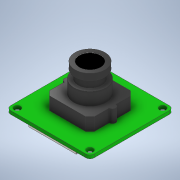
# Autodesk Inventor part: Innomaker_OV9281
Saved by Autodesk Inventor 2020 (Build 240168000, 168)
## iProperties
Created: 2021-04-16
Part Number: Innomaker_OV9281
Material: Generic
Document SubType Name: Modeling
Designer: junnu
Density: 1 g/cm^3
Appearance: Default
Author: junnu
Autodesk Inventor part; units mm, degrees
ref_plane "YZ Plane" through (0, 0, 0) normal (1, 0, 0) x (0, 1, 0)
ref_plane "XZ Plane" through (0, 0, 0) normal (0, 1, 0) x (-1, 0, 0)
ref_plane "XY Plane" through (0, 0, 0) normal (0, 0, 1) x (1, 0, 0)
sketch "Sketch1" plane through (0, 0, 0) normal (0, 1, 0) x (-1, 0, 0)
  line L0 (17.55, 19.55) -> (-17.55, 19.55)
  line L1 (-19.55, 17.55) -> (-19.55, -17.55)
  line L2 (-17.55, -19.55) -> (17.55, -19.55)
  line L3 (19.55, -17.55) -> (19.55, 17.55)
  line L4 (19.55, 19.55) -> (-19.55, -19.55) construction
  line L5 (-19.55, 19.55) -> (19.55, -19.55) construction
  line L6 (17, 17) -> (-17, 17) construction
  line L7 (-17, 17) -> (-17, -17) construction
  line L8 (-17, -17) -> (17, -17) construction
  line L9 (17, -17) -> (17, 17) construction
  line L10 (17, 17) -> (-17, -17) construction
  line L11 (-17, 17) -> (17, -17) construction
  circle A0 centre (17, -17) radius 1.5
  circle A1 centre (-17, -17) radius 1.5
  circle A2 centre (17, 17) radius 1.5
  circle A3 centre (-17, 17) radius 1.5
  arc A4 (17.55, -19.55) -> (19.55, -17.55) centre (17.55, -17.55) ccw
  arc A5 (-19.55, -17.55) -> (-17.55, -19.55) centre (-17.55, -17.55) ccw
  arc A6 (-17.55, 19.55) -> (-19.55, 17.55) centre (-17.55, 17.55) ccw
  arc A7 (19.55, 17.55) -> (17.55, 19.55) centre (17.55, 17.55) ccw
  point P0 (0, 0)
  dimension "d0" = 39.1
  dimension "d1" = 39.1
  dimension "d2" = 34
  dimension "d3" = 34
  dimension "d4" = 3
  dimension "d5" = 3
  dimension "d6" = 3
  dimension "d7" = 3
  dimension "d8" = 2
  constraints: 24 end point, 8 centre point, 8 point on circle, 8 point on line, 8 tangent, 4 coincident, 4 midpoint, 4 parallel, 3 equal radius, 2 horizontal, 2 perpendicular
  measures "d0" distance of L5.end L4.end
  measures "d1" distance of L4.end L5.start
  measures "d2" distance of L8.end L7.end
  measures "d3" distance of L7.end L6.end
  measures "d4" diameter of A0
  measures "d5" diameter of A1
  measures "d6" diameter of A2
  measures "d7" diameter of A3
  measures "d8" radius of A4
extrude "Extrusion1" add sketch "Sketch1" along normal blind 1.6
sketch "Sketch2" plane through (0, 1.6, 0) normal (0, 1, 0) x (1, 0, 0)
  line L0 (-8.5, -10.5) -> (8.5, -10.5)
  line L1 (10.5, -8.5) -> (10.5, 8.5)
  line L2 (8.5, 10.5) -> (-8.5, 10.5)
  line L3 (-10.5, 8.5) -> (-10.5, -8.5)
  line L4 (-10.5, -10.5) -> (10.5, 10.5) construction
  line L5 (10.5, -10.5) -> (-10.5, 10.5) construction
  line L6 (-8.5, 10.5) -> (-10.5, 8.5)
  line L7 (8.5, 10.5) -> (10.5, 8.5)
  line L8 (8.5, -10.5) -> (10.5, -8.5)
  line L9 (-8.5, -10.5) -> (-10.5, -8.5)
  circle A0 centre (-10.5, 0) radius 1.5
  circle A1 centre (10.5, 0) radius 1.5
  point P0 (0, 0)
  point P1 (10.5, 1.5)
  point P2 (-10.5, 1.5)
  point P3 (-10.5, -1.5)
  point P4 (10.5, -1.5)
  dimension "d11" = 21
  dimension "d12" = 21
  dimension "d13" = 2
  dimension "d14" = 2
  dimension "d15" = 2
  dimension "d16" = 2
  dimension "d17" = 2
  dimension "d18" = 2
  dimension "d19" = 2
  dimension "d20" = 2
  dimension "d21" = 3
  dimension "d22" = 3
  constraints: 20 end point, 8 point on line, 4 midpoint, 2 centre point, 2 parallel, 1 horizontal, 1 perpendicular
  measures "d11" distance of L5.end L4.end
  measures "d12" distance of L4.end L5.start
  measures "d13" distance of L2.end L5.end
  measures "d14" distance of L3.start L5.end
  measures "d15" distance of L2.start L4.end
  measures "d16" distance of L1.end L4.end
  measures "d17" distance of L0.end L5.start
  measures "d18" distance of L1.start L5.start
  measures "d19" distance of L0.start L4.start
  measures "d20" distance of L3.end L4.start
  measures "d21" diameter of A0
  measures "d22" diameter of A1
extrude "Extrusion2" add sketch "Sketch2" along normal blind 6
sketch "Sketch3" plane through (0, 7.6, 0) normal (0, 1, 0) x (1, 0, 0)
  circle A0 centre (0, 0) radius 7.5
  dimension "d25" = 15
  constraints: 1 centre point, 1 coincident
  measures "d25" diameter of A0
extrude "Extrusion3" add sketch "Sketch3" along normal blind 6
sketch "Sketch4" plane through (0, 13.6, 0) normal (0, 1, 0) x (1, 0, 0)
  circle A0 centre (0, 0) radius 5.5
  dimension "d28" = 11
  constraints: 1 centre point, 1 coincident
  measures "d28" diameter of A0
extrude "Extrusion4" add sketch "Sketch4" along normal blind 4
sketch "Sketch5" plane through (0, 17.6, 0) normal (0, 1, 0) x (1, 0, 0)
  circle A0 centre (0, 0) radius 7
  dimension "d31" = 14
  constraints: 1 centre point, 1 coincident
  measures "d31" diameter of A0
extrude "Extrusion5" add sketch "Sketch5" along normal blind 3
sketch "Sketch6" plane through (0, 20.6, 0) normal (0, 1, 0) x (1, 0, 0)
  circle A0 centre (0, 0) radius 5
  dimension "d34" = 10
  constraints: 1 centre point, 1 coincident
  measures "d34" diameter of A0
extrude "Extrusion6" cut sketch "Sketch6" against normal blind 0.2
sketch "Sketch7" plane through (0, 0, 0) normal (0, -1, 0) x (1, 0, 0)
  arc A0 (10.5, -1.5) -> (10.5, 1.5) centre (10.5, 0) ccw construction
  arc A1 (-10.5, 1.5) -> (-10.5, -1.5) centre (-10.5, 0) ccw construction
  circle A2 centre (10.5, 0) radius 1
  circle A3 centre (-10.5, 0) radius 1
  point P0 (0, 0)
  dimension "d37" = 2
  dimension "d38" = 2
  constraints: 2 centre point, 2 coincident
  measures "d37" diameter of A2
  measures "d38" diameter of A3
extrude "Extrusion7" cut sketch "Sketch7" against normal blind 5
sketch "Sketch8" plane through (0, 0, 0) normal (0, -1, 0) x (1, 0, 0)
  circle A0 centre (10.5, 0) radius 1 construction
  circle A1 centre (-10.5, 0) radius 1 construction
  arc A2 (17.55, -19.55) -> (19.55, -17.55) centre (17.55, -17.55) ccw construction
  line L0 (19.55, 17.55) -> (19.55, -17.55) construction
  arc A3 (19.55, 17.55) -> (17.55, 19.55) centre (17.55, 17.55) ccw construction
  line L1 (-17.55, 19.55) -> (17.55, 19.55) construction
  arc A4 (-17.55, 19.55) -> (-19.55, 17.55) centre (-17.55, 17.55) ccw construction
  line L2 (-19.55, -17.55) -> (-19.55, 17.55) construction
  arc A5 (-19.55, -17.55) -> (-17.55, -19.55) centre (-17.55, -17.55) ccw construction
  line L3 (17.55, -19.55) -> (-17.55, -19.55) construction
  circle A6 centre (17, -17) radius 1.5 construction
  circle A7 centre (17, 17) radius 1.5 construction
  circle A8 centre (-17, -17) radius 1.5 construction
  circle A9 centre (-17, 17) radius 1.5 construction
  line L4 (-17.55, 19.55) -> (17.55, 19.55) construction
  line L5 (0, 19.55) -> (0, 17.55) construction
  line L6 (0, 17.55) -> (0, 12.2) construction
  line L7 (11.09, 17.55) -> (-11.09, 17.55)
  line L8 (-11.09, 17.55) -> (-11.09, 12.2)
  line L9 (-11.09, 12.2) -> (11.09, 12.2)
  line L10 (11.09, 12.2) -> (11.09, 17.55)
  line L11 (11.09, 17.55) -> (-11.09, 12.2) construction
  line L12 (-11.09, 17.55) -> (11.09, 12.2) construction
  point P0 (0, 0)
  point P1 (0, 14.875)
  dimension "d41" = 2
  dimension "d42" = 5.35
  dimension "d43" = 22.18
  dimension "d44" = 5.35
  constraints: 16 end point, 4 midpoint, 2 parallel, 2 vertical, 1 horizontal, 1 perpendicular
  measures "d41" distance of L5.start L5.end
  measures "d42" distance of L5.end L6.end
  measures "d43" distance of L9.end L8.end
  measures "d44" distance of L8.end L7.end
extrude "Extrusion8" add sketch "Sketch8" along normal blind 2.8
equation "\"d14\" = d13"
equation "\"d15\" = d13"
equation "\"d16\" = d15"
equation "\"d17\" = d13"
equation "\"d18\" = d17"
equation "\"d19\" = d13"
equation "\"d20\" = d19"
body "Solid1"
